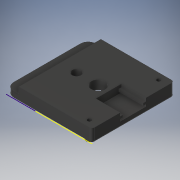
# Autodesk Inventor part: Microscopio Sujetador de
Saved by Autodesk Inventor 2018 (Build 220112000, 112)
## iProperties
Created: 2018-04-17
Part Number: Microscopio Sujetador de
Material: Thermoplastic Resin
Document SubType Name: Modeling
Designer: dm0814
Density: 1.28 g/cm^3
Appearance: Smooth - Black
Author: dm0814
Autodesk Inventor part; units mm, degrees
ref_plane "YZ Plane" through (0, 0, 0) normal (1, 0, 0) x (0, 1, 0)
ref_plane "XZ Plane" through (0, 0, 0) normal (0, 1, 0) x (-1, 0, 0)
ref_plane "XY Plane" through (0, 0, 0) normal (0, 0, 1) x (1, 0, 0)
sketch "Sketch1" plane through (0, 0, 0) normal (0, 0, 1) x (1, 0, 0)
  line L0 (0, 0) -> (67, 0)
  line L1 (67, 0) -> (67, 64)
  line L2 (67, 64) -> (0, 64)
  line L3 (0, 64) -> (0, 0)
  dimension "d0" = 67
  dimension "d1" = 64
  constraints: 8 end point, 2 parallel, 1 horizontal, 1 perpendicular
  measures "d0" distance of L2.end L1.end
  measures "d1" distance of L1.end L0.end
extrude "Extrusion1" add sketch "Sketch1" along normal blind 10
sketch "Sketch2" plane through (0, 0, 10) normal (0, 0, 1) x (1, 0, 0)
  line L0 (67, 64) -> (0, 64) projected
  line L1 (0, 0) -> (67, 0) projected
  line L2 (0, 64) -> (10, 64)
  line L3 (10, 64) -> (10, 0)
  line L4 (10, 0) -> (0, 0)
  line L5 (0, 0) -> (0, 64)
  dimension "d4" = 10
  constraints: 8 end point, 2 parallel, 1 horizontal, 1 perpendicular, 1 point on line
  measures "d4" distance of L3.end L4.end
extrude "Extrusion2" cut sketch "Sketch2" against normal blind 5
sketch "Sketch3" plane through (0, 0, 0) normal (0, 0, -1) x (-1, 0, 0)
  line L0 (0, 0) -> (-67, 0) projected
  line L1 (0, 0) -> (0, 32)
  line L2 (0, 64) -> (0, 0) projected
  line L3 (0, 32) -> (-23, 32)
  circle A0 centre (-23, 32) radius 3.5
  dimension "d7" = 23
  dimension "d8" = 7
  constraints: 4 end point, 1 centre point, 1 coincident, 1 midpoint, 1 perpendicular
  measures "d7" distance of L1.end L3.end
  measures "d8" diameter of A0
extrude "Extrusion3" cut sketch "Sketch3" against normal blind 10
sketch "Sketch4" plane through (0, 0, 0) normal (0, 0, -1) x (-1, 0, 0)
  line L0 (0, 64) -> (0, 0) projected
  line L1 (0, 0) -> (0, 32)
  line L2 (0, 32) -> (-23, 32)
  circle A0 centre (-23, 32) radius 25
  dimension "d11" = 23
  dimension "d12" = 50
  constraints: 4 end point, 1 centre point, 1 coincident, 1 midpoint, 1 perpendicular
  measures "d11" distance of L1.end L2.end
  measures "d12" diameter of A0
extrude "Extrusion4" cut sketch "Sketch4" against normal blind 3
sketch "Sketch5" plane through (0, 0, 3) normal (0, 0, -1) x (-1, 0, 0)
  line L0 (0, 0) -> (0, 64) projected
  line L1 (0, 0) -> (0, 32)
  line L2 (0, 32) -> (-34.5, 32)
  line L3 (-34.5, 32) -> (-40, 32)
  circle A0 centre (-40, 32) radius 5.5
  dimension "d15" = 34.5
  dimension "d16" = 5.5
  dimension "d17" = 11
  constraints: 6 end point, 1 centre point, 1 coincident, 1 horizontal, 1 midpoint, 1 point on line
  measures "d15" distance of L1.end L2.end
  measures "d16" distance of L2.end L3.end
  measures "d17" diameter of A0
extrude "Extrusion5" cut sketch "Sketch5" against normal blind 10
sketch "Sketch6" plane through (0, 0, 0) normal (0, 0, -1) x (-1, 0, 0)
  line L0 (0, 0) -> (-67, 0) projected
  line L1 (-67, 0) -> (-67, 32)
  line L2 (-67, 0) -> (-67, 64) projected
  line L3 (-67, 32) -> (-66, 32)
  line L4 (-66, 32) -> (-66, 23.5)
  line L5 (-66, 23.5) -> (-53, 23.5)
  line L6 (-53, 23.5) -> (-53, 40.5)
  line L7 (-53, 40.5) -> (-66, 40.5)
  line L8 (-66, 40.5) -> (-66, 23.5)
  dimension "d20" = 1
  dimension "d21" = 8.5
  dimension "d22" = 13
  dimension "d23" = 17
  constraints: 14 end point, 2 parallel, 2 perpendicular, 1 horizontal, 1 midpoint, 1 vertical
  measures "d20" distance of L1.end L3.end
  measures "d21" distance of L3.end L4.end
  measures "d22" distance of L7.end L6.end
  measures "d23" distance of L6.end L5.end
extrude "Extrusion6" cut sketch "Sketch6" against normal blind 2
sketch "Sketch7" plane through (0, 0, 0) normal (0, 0, -1) x (-1, 0, 0)
  line L0 (0, 0) -> (-23, 0)
  line L1 (0, 0) -> (-67, 0) projected
  constraints: 2 end point, 1 point on line
sketch "Sketch8" plane through (0, 0, 0) normal (0, 0, -1) x (-1, 0, 0)
  line L0 (-23, 1) -> (-11.75, 1)
  line L1 (-11.75, 1) -> (-34.25, 1)
  line L2 (-34.25, 3.5) -> (-11.75, 3.5)
  line L3 (0, 64) -> (0, 41.798) projected
  line L4 (0, 64) -> (-23, 64)
  line L5 (-67, 64) -> (-10, 64) projected
  line L6 (-23, 63) -> (-34.25, 63)
  line L7 (-34.25, 63) -> (-11.75, 63)
  line L8 (-11.75, 60.5) -> (-34.25, 60.5)
  arc A0 (-11.75, 1) -> (-11.75, 3.5) centre (-11.75, 2.25) ccw
  arc A1 (-34.25, 3.5) -> (-34.25, 1) centre (-34.25, 2.25) ccw
  arc A2 (-11.75, 60.5) -> (-11.75, 63) centre (-11.75, 61.75) ccw
  arc A3 (-34.25, 63) -> (-34.25, 60.5) centre (-34.25, 61.75) ccw
  point P0 (0, 0)
  constraints: 14 end point, 8 point on circle, 4 centre point, 2 horizontal, 2 parallel, 1 point on line
extrude "Extrusion7" cut sketch "Sketch8" against normal blind 3
sketch "Sketch9" plane through (0, 0, 0) normal (0, 0, -1) x (-1, 0, 0)
  line L0 (-67, 0) -> (-67, 64) projected
  line L1 (-67, 64) -> (-60, 64)
  line L2 (-67, 64) -> (-10, 64) projected
  line L3 (-60, 64) -> (-60, 59)
  line L4 (-10, 0) -> (-67, 0) projected
  line L5 (-67, 0) -> (-60, 0)
  line L6 (-60, 0) -> (-60, 5)
  circle A0 centre (-60, 59) radius 2.5
  circle A1 centre (-60, 5) radius 2.5
  point P0 (0, 0)
  dimension "d55" = 7
  dimension "d56" = 5
  dimension "d57" = 7
  dimension "d58" = 5
  dimension "d59" = 5
  dimension "d60" = 5
  constraints: 8 end point, 2 centre point, 2 coincident, 2 perpendicular, 2 point on line
  measures "d55" distance of L0.end L1.end
  measures "d56" distance of L1.end L3.end
  measures "d57" distance of L0.start L5.end
  measures "d58" distance of L5.end L6.end
  measures "d59" diameter of A0
  measures "d60" diameter of A1
extrude "Extrusion8" add sketch "Sketch9" along normal blind 3
sketch "Sketch10" plane through (60, 5, -3) normal (0, 0, -1) x (-1, 0, 0)
  circle A0 centre (0, 0) radius 2.5 projected
  circle A1 centre (0, 0) radius 1.5
  circle A2 centre (0, 54) radius 2.5 projected
  circle A3 centre (0, 54) radius 1.5
  point P0 (60, -5)
  dimension "d63" = 3
  dimension "d64" = 3
  constraints: 2 centre point, 2 coincident
  measures "d63" diameter of A1
  measures "d64" diameter of A3
extrude "Extrusion9" cut sketch "Sketch10" against normal blind 13 contours A1 | A3
fillet "Fillet1" radius 1 5 edges at (33.5, 0, 0) (67, 32, 0) (33.5, 64, 0) (0, 52.899, 0) (0, 11.101, 0)
fillet "Fillet2" radius 6 4 edges at (0.2929, 0.2929, 0.2929) (0, 0, 2.9999) (0.2929, 63.7071, 0.2929) (0, 64, 2.9999)
fillet "Fillet3" radius 2 4 edges at (66.7071, 0.2929, 0.2929) (67, 0, 5.5) (66.7071, 63.7071, 0.2929) (67, 64, 5.5)
sketch "Sketch11" plane through (67, 2, 10) normal (1, 0, 0) x (0, 0, -1)
  line L0 (0, 62) -> (0, -2) projected
  line L1 (6, 40) -> (6, 20)
  line L2 (6, 20) -> (0, 20)
  line L3 (0, 20) -> (0, 40)
  line L4 (0, 60) -> (9, 60) projected
  line L5 (0, 60) -> (9, 60) projected
  line L6 (0, 0) -> (0, 60) projected
  line L7 (9, 0) -> (0, 0) projected
  line L8 (9, 60) -> (9, 0) projected
  line L9 (0, 60) -> (9, 60) projected
  line L10 (0, 0) -> (0, 60) projected
  line L11 (9, 0) -> (0, 0) projected
  line L12 (9, 60) -> (9, 0) projected
  line L13 (0, 24.5) -> (0, 35.5) projected
  line L14 (4.5, 40) -> (2.5, 40)
  line L15 (2.5, 40) -> (2.5, 38)
  line L16 (2.5, 38) -> (4.5, 38)
  line L17 (4.5, 38) -> (4.5, 40)
  line L18 (0, 20) -> (6, 20)
  line L19 (4.5, 20) -> (2.5, 20)
  line L20 (2.5, 20) -> (2.5, 22)
  line L21 (2.5, 22) -> (4.5, 22)
  line L22 (4.5, 22) -> (4.5, 20)
  line L23 (0, 40) -> (2.5, 40)
  line L24 (4.5, 40) -> (6, 40)
  point P0 (10, -2)
  dimension "d70" = 6
  dimension "d71" = 20
  dimension "d73" = 2
  dimension "d74" = 2
  dimension "d75" = 1.5
  constraints: 28 end point, 5 parallel, 3 horizontal, 3 perpendicular, 2 point on line
  measures "d70" distance of L1.end L2.end
  measures "d71" distance of L1.start L1.end
  measures "d73" distance of L16.end L15.end
  measures "d74" distance of L15.end L14.end
  measures "d75" distance of L14.start L1.start
extrude "Extrusion10" cut sketch "Sketch11" against normal blind 19 contours L23 L15 L16 L17 L24 L1 L2 L22 L21 L20 L0
body "Solid1"
